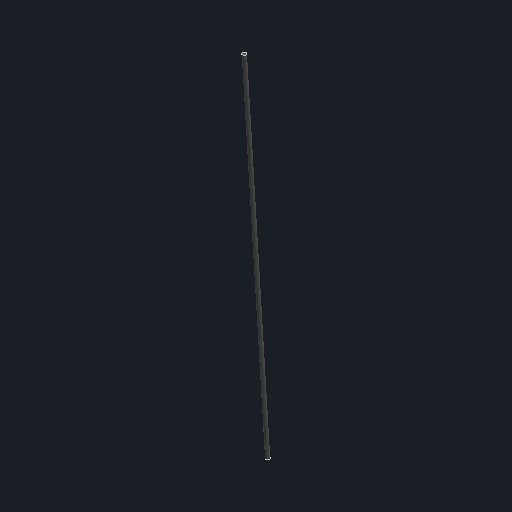
# Autodesk Inventor part: steering_rod
Saved by Autodesk Inventor 2024 (Build 280153000, 153)
## iProperties
Created: 2022-03-30
Part Number: steering_rod
Material: Generic
Document SubType Name: Modeling
Designer: kardo
Density: 1 g/cm^3
Appearance: Dark Plastic
Mass: 0.682366 g
Surface Area: 13.7101 cm^2
Volume: 0.682366 cm^3
Author: kardo
Autodesk Inventor part; units mm, degrees
ref_plane "YZ Plane" through (0, 0, 0) normal (1, 0, 0) x (0, 1, 0)
ref_plane "XZ Plane" through (0, 0, 0) normal (0, 1, 0) x (-1, 0, 0)
ref_plane "XY Plane" through (0, 0, 0) normal (0, 0, 1) x (1, 0, 0)
derived "stencil_frame.ipt"
sketch3d "sk_servo_rod"
ref_plane "Work Plane1" through (-9.6, -194.6817, 43.1496) normal (-0.0367367, -0.9944644, -0.0984426) x (0.9993184, -0.036916, 0)
sketch "Sketch1" plane through (-9.6, -194.6817, 43.1496) normal (-0.0367367, -0.9944644, -0.0984426) x (0.9993184, -0.036916, 0)
  circle A0 centre (0, 0) radius 1
  point P0 (2.4066, -62.1268)
  point P1 (0, 0)
  dimension "d1" = 2
  constraints: 1 centre point, 1 coincident
  measures "d1" diameter of A0
extrude "Extrusion1" add sketch "Sketch1" along normal up to surface (201.4333 mm away)
body "Solid1"
